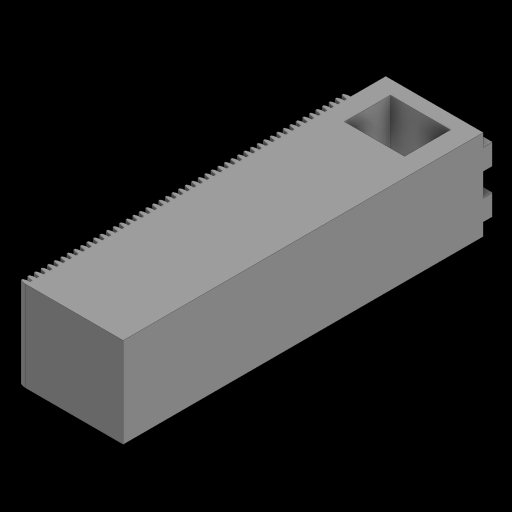
# Autodesk Inventor part: 렉기어
Saved by Autodesk Inventor 2023 (Build 270158000, 158)
## iProperties
Created: 2024-07-04
Part Number: 렉기어
Material: 일반
Document SubType Name: Modeling
Designer: OMS55
Density: 1 g/cm^3
Appearance: 기본값
Mass: 113.431 g
Surface Area: 254.945 cm^2
Volume: 113.431 cm^3
Author: OMS55
Autodesk Inventor part; units mm, degrees
ref_plane "YZ Plane" through (0, 0, 0) normal (1, 0, 0) x (0, 1, 0)
ref_plane "XZ Plane" through (0, 0, 0) normal (0, 1, 0) x (-1, 0, 0)
ref_plane "XY Plane" through (0, 0, 0) normal (0, 0, 1) x (1, 0, 0)
sketch "스케치1" plane through (0, 0, 0) normal (0, 1, 0) x (-1, 0, 0)
  line L0 (0, 0) -> (-34.5, 0)
  line L1 (-34.5, 0) -> (-34.5, -120)
  line L2 (-34.5, -120) -> (0, -120)
  line L3 (0, -120) -> (0, 0)
  line L4 (-2, 0) -> (-34.5, 0)
  line L5 (-34.5, 0) -> (-34.5, -120)
  line L6 (-34.5, -120) -> (-2, -120)
  line L7 (-2, -120) -> (-2, 0)
  arc A0 (0, -0.477) -> (-2, 0) centre (-2, -4.4314) ccw
  arc A1 (-2, -1.454) -> (0, -0.977) centre (-2, 2.9774) ccw
  line L8 (-2, -0.727) -> (0, -0.727) construction
  line L9 (0, -0.477) -> (0, -0.977)
  line L10 (-2, 0) -> (-2, -1.454)
  arc A2 (0, -2.658) -> (-2, -2.181) centre (-2, -6.6124) ccw
  line L11 (0, -2.658) -> (0, -3.158)
  arc A3 (-2, -3.635) -> (0, -3.158) centre (-2, 0.7964) ccw
  line L12 (-2, -2.181) -> (-2, -3.635)
  arc A4 (0, -4.839) -> (-2, -4.362) centre (-2, -8.7934) ccw
  line L13 (0, -4.839) -> (0, -5.339)
  arc A5 (-2, -5.816) -> (0, -5.339) centre (-2, -1.3846) ccw
  line L14 (-2, -4.362) -> (-2, -5.816)
  arc A6 (0, -7.02) -> (-2, -6.543) centre (-2, -10.9744) ccw
  line L15 (0, -7.02) -> (0, -7.52)
  arc A7 (-2, -7.997) -> (0, -7.52) centre (-2, -3.5656) ccw
  line L16 (-2, -6.543) -> (-2, -7.997)
  arc A8 (0, -9.201) -> (-2, -8.724) centre (-2, -13.1554) ccw
  line L17 (0, -9.201) -> (0, -9.701)
  arc A9 (-2, -10.178) -> (0, -9.701) centre (-2, -5.7466) ccw
  line L18 (-2, -8.724) -> (-2, -10.178)
  arc A10 (0, -11.382) -> (-2, -10.905) centre (-2, -15.3364) ccw
  line L19 (0, -11.382) -> (0, -11.882)
  arc A11 (-2, -12.359) -> (0, -11.882) centre (-2, -7.9276) ccw
  line L20 (-2, -10.905) -> (-2, -12.359)
  arc A12 (0, -13.563) -> (-2, -13.086) centre (-2, -17.5174) ccw
  line L21 (0, -13.563) -> (0, -14.063)
  arc A13 (-2, -14.54) -> (0, -14.063) centre (-2, -10.1086) ccw
  line L22 (-2, -13.086) -> (-2, -14.54)
  arc A14 (0, -15.744) -> (-2, -15.267) centre (-2, -19.6984) ccw
  line L23 (0, -15.744) -> (0, -16.244)
  arc A15 (-2, -16.721) -> (0, -16.244) centre (-2, -12.2896) ccw
  line L24 (-2, -15.267) -> (-2, -16.721)
  arc A16 (0, -17.925) -> (-2, -17.448) centre (-2, -21.8794) ccw
  line L25 (0, -17.925) -> (0, -18.425)
  arc A17 (-2, -18.902) -> (0, -18.425) centre (-2, -14.4706) ccw
  line L26 (-2, -17.448) -> (-2, -18.902)
  arc A18 (0, -20.106) -> (-2, -19.629) centre (-2, -24.0604) ccw
  line L27 (0, -20.106) -> (0, -20.606)
  arc A19 (-2, -21.083) -> (0, -20.606) centre (-2, -16.6516) ccw
  line L28 (-2, -19.629) -> (-2, -21.083)
  arc A20 (0, -22.287) -> (-2, -21.81) centre (-2, -26.2414) ccw
  line L29 (0, -22.287) -> (0, -22.787)
  arc A21 (-2, -23.264) -> (0, -22.787) centre (-2, -18.8326) ccw
  line L30 (-2, -21.81) -> (-2, -23.264)
  arc A22 (0, -24.468) -> (-2, -23.991) centre (-2, -28.4224) ccw
  line L31 (0, -24.468) -> (0, -24.968)
  arc A23 (-2, -25.445) -> (0, -24.968) centre (-2, -21.0136) ccw
  line L32 (-2, -23.991) -> (-2, -25.445)
  arc A24 (0, -26.649) -> (-2, -26.172) centre (-2, -30.6034) ccw
  line L33 (0, -26.649) -> (0, -27.149)
  arc A25 (-2, -27.626) -> (0, -27.149) centre (-2, -23.1946) ccw
  line L34 (-2, -26.172) -> (-2, -27.626)
  arc A26 (0, -28.83) -> (-2, -28.353) centre (-2, -32.7844) ccw
  line L35 (0, -28.83) -> (0, -29.33)
  arc A27 (-2, -29.807) -> (0, -29.33) centre (-2, -25.3756) ccw
  line L36 (-2, -28.353) -> (-2, -29.807)
  arc A28 (0, -31.011) -> (-2, -30.534) centre (-2, -34.9654) ccw
  line L37 (0, -31.011) -> (0, -31.511)
  arc A29 (-2, -31.988) -> (0, -31.511) centre (-2, -27.5566) ccw
  line L38 (-2, -30.534) -> (-2, -31.988)
  arc A30 (0, -33.192) -> (-2, -32.715) centre (-2, -37.1464) ccw
  line L39 (0, -33.192) -> (0, -33.692)
  arc A31 (-2, -34.169) -> (0, -33.692) centre (-2, -29.7376) ccw
  line L40 (-2, -32.715) -> (-2, -34.169)
  arc A32 (0, -35.373) -> (-2, -34.896) centre (-2, -39.3274) ccw
  line L41 (0, -35.373) -> (0, -35.873)
  arc A33 (-2, -36.35) -> (0, -35.873) centre (-2, -31.9186) ccw
  line L42 (-2, -34.896) -> (-2, -36.35)
  arc A34 (0, -37.554) -> (-2, -37.077) centre (-2, -41.5084) ccw
  line L43 (0, -37.554) -> (0, -38.054)
  arc A35 (-2, -38.531) -> (0, -38.054) centre (-2, -34.0996) ccw
  line L44 (-2, -37.077) -> (-2, -38.531)
  arc A36 (0, -39.735) -> (-2, -39.258) centre (-2, -43.6894) ccw
  line L45 (0, -39.735) -> (0, -40.235)
  arc A37 (-2, -40.712) -> (0, -40.235) centre (-2, -36.2806) ccw
  line L46 (-2, -39.258) -> (-2, -40.712)
  arc A38 (0, -41.916) -> (-2, -41.439) centre (-2, -45.8704) ccw
  line L47 (0, -41.916) -> (0, -42.416)
  arc A39 (-2, -42.893) -> (0, -42.416) centre (-2, -38.4616) ccw
  line L48 (-2, -41.439) -> (-2, -42.893)
  arc A40 (0, -44.097) -> (-2, -43.62) centre (-2, -48.0514) ccw
  line L49 (0, -44.097) -> (0, -44.597)
  arc A41 (-2, -45.074) -> (0, -44.597) centre (-2, -40.6426) ccw
  line L50 (-2, -43.62) -> (-2, -45.074)
  arc A42 (0, -46.278) -> (-2, -45.801) centre (-2, -50.2324) ccw
  line L51 (0, -46.278) -> (0, -46.778)
  arc A43 (-2, -47.255) -> (0, -46.778) centre (-2, -42.8236) ccw
  line L52 (-2, -45.801) -> (-2, -47.255)
  arc A44 (0, -48.459) -> (-2, -47.982) centre (-2, -52.4134) ccw
  line L53 (0, -48.459) -> (0, -48.959)
  arc A45 (-2, -49.436) -> (0, -48.959) centre (-2, -45.0046) ccw
  line L54 (-2, -47.982) -> (-2, -49.436)
  arc A46 (0, -50.64) -> (-2, -50.163) centre (-2, -54.5944) ccw
  line L55 (0, -50.64) -> (0, -51.14)
  arc A47 (-2, -51.617) -> (0, -51.14) centre (-2, -47.1856) ccw
  line L56 (-2, -50.163) -> (-2, -51.617)
  arc A48 (0, -52.821) -> (-2, -52.344) centre (-2, -56.7754) ccw
  line L57 (0, -52.821) -> (0, -53.321)
  arc A49 (-2, -53.798) -> (0, -53.321) centre (-2, -49.3666) ccw
  line L58 (-2, -52.344) -> (-2, -53.798)
  arc A50 (0, -55.002) -> (-2, -54.525) centre (-2, -58.9564) ccw
  line L59 (0, -55.002) -> (0, -55.502)
  arc A51 (-2, -55.979) -> (0, -55.502) centre (-2, -51.5476) ccw
  line L60 (-2, -54.525) -> (-2, -55.979)
  arc A52 (0, -57.183) -> (-2, -56.706) centre (-2, -61.1374) ccw
  line L61 (0, -57.183) -> (0, -57.683)
  arc A53 (-2, -58.16) -> (0, -57.683) centre (-2, -53.7286) ccw
  line L62 (-2, -56.706) -> (-2, -58.16)
  arc A54 (0, -59.364) -> (-2, -58.887) centre (-2, -63.3184) ccw
  line L63 (0, -59.364) -> (0, -59.864)
  arc A55 (-2, -60.341) -> (0, -59.864) centre (-2, -55.9096) ccw
  line L64 (-2, -58.887) -> (-2, -60.341)
  arc A56 (0, -61.545) -> (-2, -61.068) centre (-2, -65.4994) ccw
  line L65 (0, -61.545) -> (0, -62.045)
  arc A57 (-2, -62.522) -> (0, -62.045) centre (-2, -58.0906) ccw
  line L66 (-2, -61.068) -> (-2, -62.522)
  arc A58 (0, -63.726) -> (-2, -63.249) centre (-2, -67.6804) ccw
  line L67 (0, -63.726) -> (0, -64.226)
  arc A59 (-2, -64.703) -> (0, -64.226) centre (-2, -60.2716) ccw
  line L68 (-2, -63.249) -> (-2, -64.703)
  arc A60 (0, -65.907) -> (-2, -65.43) centre (-2, -69.8614) ccw
  line L69 (0, -65.907) -> (0, -66.407)
  arc A61 (-2, -66.884) -> (0, -66.407) centre (-2, -62.4526) ccw
  line L70 (-2, -65.43) -> (-2, -66.884)
  arc A62 (0, -68.088) -> (-2, -67.611) centre (-2, -72.0424) ccw
  line L71 (0, -68.088) -> (0, -68.588)
  arc A63 (-2, -69.065) -> (0, -68.588) centre (-2, -64.6336) ccw
  line L72 (-2, -67.611) -> (-2, -69.065)
  arc A64 (0, -70.269) -> (-2, -69.792) centre (-2, -74.2234) ccw
  line L73 (0, -70.269) -> (0, -70.769)
  arc A65 (-2, -71.246) -> (0, -70.769) centre (-2, -66.8146) ccw
  line L74 (-2, -69.792) -> (-2, -71.246)
  arc A66 (0, -72.45) -> (-2, -71.973) centre (-2, -76.4044) ccw
  line L75 (0, -72.45) -> (0, -72.95)
  arc A67 (-2, -73.427) -> (0, -72.95) centre (-2, -68.9956) ccw
  line L76 (-2, -71.973) -> (-2, -73.427)
  arc A68 (0, -74.631) -> (-2, -74.154) centre (-2, -78.5854) ccw
  line L77 (0, -74.631) -> (0, -75.131)
  arc A69 (-2, -75.608) -> (0, -75.131) centre (-2, -71.1766) ccw
  line L78 (-2, -74.154) -> (-2, -75.608)
  arc A70 (0, -76.812) -> (-2, -76.335) centre (-2, -80.7664) ccw
  line L79 (0, -76.812) -> (0, -77.312)
  arc A71 (-2, -77.789) -> (0, -77.312) centre (-2, -73.3576) ccw
  line L80 (-2, -76.335) -> (-2, -77.789)
  arc A72 (0, -78.993) -> (-2, -78.516) centre (-2, -82.9474) ccw
  line L81 (0, -78.993) -> (0, -79.493)
  arc A73 (-2, -79.97) -> (0, -79.493) centre (-2, -75.5386) ccw
  line L82 (-2, -78.516) -> (-2, -79.97)
  arc A74 (0, -81.174) -> (-2, -80.697) centre (-2, -85.1284) ccw
  line L83 (0, -81.174) -> (0, -81.674)
  arc A75 (-2, -82.151) -> (0, -81.674) centre (-2, -77.7196) ccw
  line L84 (-2, -80.697) -> (-2, -82.151)
  arc A76 (0, -83.355) -> (-2, -82.878) centre (-2, -87.3094) ccw
  line L85 (0, -83.355) -> (0, -83.855)
  arc A77 (-2, -84.332) -> (0, -83.855) centre (-2, -79.9006) ccw
  line L86 (-2, -82.878) -> (-2, -84.332)
  arc A78 (0, -85.536) -> (-2, -85.059) centre (-2, -89.4904) ccw
  line L87 (0, -85.536) -> (0, -86.036)
  arc A79 (-2, -86.513) -> (0, -86.036) centre (-2, -82.0816) ccw
  line L88 (-2, -85.059) -> (-2, -86.513)
  arc A80 (0, -87.717) -> (-2, -87.24) centre (-2, -91.6714) ccw
  line L89 (0, -87.717) -> (0, -88.217)
  arc A81 (-2, -88.694) -> (0, -88.217) centre (-2, -84.2626) ccw
  line L90 (-2, -87.24) -> (-2, -88.694)
  arc A82 (0, -89.898) -> (-2, -89.421) centre (-2, -93.8524) ccw
  line L91 (0, -89.898) -> (0, -90.398)
  arc A83 (-2, -90.875) -> (0, -90.398) centre (-2, -86.4436) ccw
  line L92 (-2, -89.421) -> (-2, -90.875)
  arc A84 (0, -92.079) -> (-2, -91.602) centre (-2, -96.0334) ccw
  line L93 (0, -92.079) -> (0, -92.579)
  arc A85 (-2, -93.056) -> (0, -92.579) centre (-2, -88.6246) ccw
  line L94 (-2, -91.602) -> (-2, -93.056)
  arc A86 (0, -94.26) -> (-2, -93.783) centre (-2, -98.2144) ccw
  line L95 (0, -94.26) -> (0, -94.76)
  arc A87 (-2, -95.237) -> (0, -94.76) centre (-2, -90.8056) ccw
  line L96 (-2, -93.783) -> (-2, -95.237)
  arc A88 (0, -96.441) -> (-2, -95.964) centre (-2, -100.3954) ccw
  line L97 (0, -96.441) -> (0, -96.941)
  arc A89 (-2, -97.418) -> (0, -96.941) centre (-2, -92.9866) ccw
  line L98 (-2, -95.964) -> (-2, -97.418)
  arc A90 (0, -98.622) -> (-2, -98.145) centre (-2, -102.5764) ccw
  line L99 (0, -98.622) -> (0, -99.122)
  arc A91 (-2, -99.599) -> (0, -99.122) centre (-2, -95.1676) ccw
  line L100 (-2, -98.145) -> (-2, -99.599)
  arc A92 (0, -100.803) -> (-2, -100.326) centre (-2, -104.7574) ccw
  line L101 (0, -100.803) -> (0, -101.303)
  arc A93 (-2, -101.78) -> (0, -101.303) centre (-2, -97.3486) ccw
  line L102 (-2, -100.326) -> (-2, -101.78)
  arc A94 (0, -102.984) -> (-2, -102.507) centre (-2, -106.9384) ccw
  line L103 (0, -102.984) -> (0, -103.484)
  arc A95 (-2, -103.961) -> (0, -103.484) centre (-2, -99.5296) ccw
  line L104 (-2, -102.507) -> (-2, -103.961)
  arc A96 (0, -105.165) -> (-2, -104.688) centre (-2, -109.1194) ccw
  line L105 (0, -105.165) -> (0, -105.665)
  arc A97 (-2, -106.142) -> (0, -105.665) centre (-2, -101.7106) ccw
  line L106 (-2, -104.688) -> (-2, -106.142)
  arc A98 (0, -107.346) -> (-2, -106.869) centre (-2, -111.3004) ccw
  line L107 (0, -107.346) -> (0, -107.846)
  arc A99 (-2, -108.323) -> (0, -107.846) centre (-2, -103.8916) ccw
  line L108 (-2, -106.869) -> (-2, -108.323)
  point P0 (-2, -84.332)
  point P1 (0, -83.355)
  point P2 (-2, -60.341)
  point P3 (0, -59.364)
  point P4 (-2, -58.887)
  point P5 (-2, -108.323)
  point P6 (0, -107.346)
  point P7 (-2, -106.142)
  point P8 (0, -105.165)
  point P9 (-2, -103.961)
  point P10 (0, -102.984)
  point P11 (-2, -101.78)
  point P12 (0, -100.803)
  point P13 (-2, -99.599)
  point P14 (0, -98.622)
  point P15 (-2, -97.418)
  point P16 (0, -96.441)
  point P17 (-2, -95.237)
  point P18 (0, -94.26)
  point P19 (-2, -93.056)
  point P20 (0, -92.079)
  point P21 (-2, -90.875)
  point P22 (0, -89.898)
  point P23 (0, -85.536)
  point P24 (-2, -88.694)
  point P25 (-2, -82.151)
  point P26 (0, -81.174)
  point P27 (-2, -79.97)
  point P28 (0, -78.993)
  point P29 (-2, -78.516)
  point P30 (-2, -77.789)
  point P31 (0, -76.812)
  point P32 (-2, -76.335)
  point P33 (-2, -75.608)
  point P34 (0, -74.631)
  point P35 (-2, -73.427)
  point P36 (0, -72.45)
  point P37 (-2, -71.246)
  point P38 (0, -70.269)
  point P39 (-2, -69.065)
  point P40 (0, -68.088)
  point P41 (-2, -66.884)
  point P42 (0, -65.907)
  point P43 (-2, -64.703)
  point P44 (0, -63.726)
  point P45 (-2, -63.249)
  point P46 (-2, -62.522)
  point P47 (0, -61.545)
  point P48 (-2, -61.068)
  point P49 (-2, -58.16)
  point P50 (0, -57.183)
  point P51 (-2, -56.706)
  point P52 (-2, -53.798)
  point P53 (0, -52.821)
  point P54 (-2, -52.344)
  point P55 (-2, -51.617)
  point P56 (0, -50.64)
  point P57 (-2, -50.163)
  point P58 (-2, -49.436)
  point P59 (0, -48.459)
  point P60 (-2, -47.982)
  point P61 (-2, -47.255)
  point P62 (0, -46.278)
  point P63 (-2, -45.801)
  point P64 (-2, -45.074)
  point P65 (0, -44.097)
  point P66 (-2, -43.62)
  point P67 (-2, -38.531)
  point P68 (0, -37.554)
  point P69 (-2, -34.169)
  point P70 (-2, -32.715)
  point P71 (-2, -29.807)
  point P72 (0, -28.83)
  point P73 (-2, -28.353)
  point P74 (-2, -25.445)
  point P75 (0, -24.468)
  point P76 (-2, -23.991)
  point P77 (-2, -23.264)
  point P78 (0, -22.287)
  point P79 (-2, -21.81)
  point P80 (-2, -55.979)
  point P81 (0, -55.002)
  point P82 (-2, -54.525)
  point P83 (-2, -42.893)
  point P84 (0, -41.916)
  point P85 (-2, -41.439)
  point P86 (-2, -40.712)
  point P87 (0, -39.735)
  point P88 (-2, -39.258)
  point P89 (-2, -36.35)
  point P90 (0, -35.373)
  point P91 (-2, -31.988)
  point P92 (-2, -30.534)
  point P93 (-2, -27.626)
  point P94 (0, -26.649)
  point P95 (-2, -26.172)
  point P96 (-2, -21.083)
  point P97 (0, -20.106)
  point P98 (-2, -19.629)
  point P99 (-2, -18.902)
  point P100 (-2, -16.721)
  point P101 (-2, -14.54)
  point P102 (0, -13.563)
  point P103 (-2, -12.359)
  point P104 (0, -11.382)
  point P105 (-2, -10.178)
  point P106 (-2, -7.997)
  point P107 (0, -7.02)
  point P108 (-2, -5.816)
  point P109 (0, -4.839)
  point P110 (-2, -4.362)
  point P111 (-2, -3.635)
  point P112 (0, -2.658)
  point P113 (-2, -2.181)
  point P114 (0, -87.717)
  point P115 (-2, -86.513)
  dimension "d0" = 120
  dimension "d1" = 34.5
  dimension "d2" = 120
  dimension "d3" = 32.5
  dimension "d4" = 1.454
  dimension "d7" = 0.727
  dimension "d8" = 0.25
  dimension "d9" = 0.25
  dimension "d14" = 2.181
  constraints: 294 vertical alignment, 214 end point, 200 point on circle, 100 centre point, 98 collinear, 98 equal radius, 4 vertical, 3 horizontal, 2 parallel, 2 perpendicular, 1 coincident, 1 tangent, 10 other
  measures "d0" distance of L2.end L0.start
  measures "d1" distance of L0.start L0.end
  measures "d2" distance of L6.end L4.start
  measures "d3" distance of L0.end L4.start
  measures "d4" distance of L10.end L4.start
  measures "d7" distance of L8.start L4.start
  measures "d8" distance of L8.end L9.start
  measures "d9" distance of L8.end L9.end
  measures "d14" distance of A0.centre A2.centre
extrude "돌출1" add sketch "스케치1" along normal blind 30 contours L7 L2 L1 L0 | A0 L3 A1 L7 | A2 L3 A3 L7 | L7 A98 L3 A99 | A4 L3 A5 L7 | L7 A96 L3 A97 | A6 L3 A7 L7 | L7 A94 L3 A95 | A8 L3 A9 L7 | L7 A92 L3 A93 | A10 L3 A11 L7 | L7 A90 L3 A91 | A12 L3 A13 L7 | L7 A88 L3 A89 | A14 L3 A15 L7 | L7 A86 L3 A87 | A16 L3 A17 L7 | L7 A84 L3 A85 | A18 L3 A19 L7 | L7 A82 L3 A83 | A20 L3 A21 L7 | L7 A80 L3 A81 | A22 L3 A23 L7 | L7 A79 L3 A80 | L7 A78 L3 A79 | A24 L3 A25 L7 | L7 A76 L3 A77 | A26 L3 A27 L7 | L7 A74 L3 A75 | A28 L3 A29 L7 | L7 A72 L3 A73 | A30 L3 A31 L7 | L7 A70 L3 A71 | A32 L3 A33 L7 | L7 A68 L3 A69 | A34 L3 A35 L7 | L7 A66 L3 A67 | A36 L3 A37 L7 | L7 A64 L3 A65 | A38 L3 A39 L7 | L7 A62 L3 A63 | A40 L3 A41 L7 | L7 A60 L3 A61 | A42 L3 A43 L7 | L7 A58 L3 A59 | A44 L3 A45 L7 | L7 A56 L3 A57 | A46 L3 A47 L7 | L7 A54 L3 A55 | A48 L3 A49 L7 | L7 A52 L3 A53 | A50 L3 A51 L7
extrude "돌출2" cut sketch "스케치1" along normal blind 30 contours L7 A79 L3 A80
sketch "스케치2" plane through (34.5, 0, -120) normal (0, 0, -1) x (-1, 0, 0)
  line L0 (32.5, 25.8) -> (0, 25.8)
  line L1 (0, 25.8) -> (0, 18.8)
  line L2 (0, 18.8) -> (32.5, 18.8)
  line L3 (32.5, 18.8) -> (32.5, 25.8)
  line L4 (32.5, 11.2) -> (0, 11.2)
  line L5 (0, 11.2) -> (0, 4.2)
  line L6 (0, 4.2) -> (32.5, 4.2)
  line L7 (32.5, 4.2) -> (32.5, 11.2)
  line L8 (32.5, 18.8) -> (32.5, 11.2) construction
  line L9 (0, 18.8) -> (0, 11.2) construction
  line L10 (32.5, 0) -> (32.5, 30) construction
  line L11 (0, 0) -> (0, 30) construction
  point P0 (34.5, 0)
  point P1 (32.5, 15)
  point P2 (32.5, 15)
  dimension "d21" = 7.6
  dimension "d22" = 7
  dimension "d23" = 7
  constraints: 20 end point, 5 parallel, 2 collinear, 2 horizontal, 2 midpoint, 2 perpendicular, 2 point on line, 1 coincident, 1 vertical
  measures "d21" distance between parallel lines of L4 L2
  measures "d22" distance of L2.end L0.start
  measures "d23" distance of L6.end L4.start
extrude "돌출3" add sketch "스케치2" along normal blind 3
sketch "스케치4" plane through (0, 30, 0) normal (0, 1, 0) x (1, 0, 0)
  line L0 (28.25, 115.3) -> (8.25, 115.3)
  line L1 (8.25, 115.3) -> (8.25, 100)
  line L2 (8.25, 100) -> (28.25, 100)
  line L3 (28.25, 100) -> (28.25, 115.3)
  line L4 (34.5, 120) -> (2, 120) projected
  line L5 (34.5, 0) -> (34.5, 120) projected
  point P0 (0, 0)
  dimension "d26" = 20
  dimension "d27" = 20
  dimension "d28" = 6.25
  dimension "d29" = 4.7
  constraints: 8 end point, 2 parallel, 1 horizontal, 1 perpendicular
  measures "d26" distance between parallel lines of L2 L4
  measures "d27" distance between parallel lines of L1 L3
  measures "d28" distance between parallel lines of L5 L3
  measures "d29" distance between parallel lines of L4 L0
extrude "돌출4" cut sketch "스케치4" against normal blind 30
sketch "스케치5" plane through (8.25, 30, -115.3) normal (0, 0, 1) x (1, 0, 0)
  circle A0 centre (7.45, -15) radius 1.45
  line L0 (-6.25, -18.8) -> (-6.25, -11.2) projected
  point P0 (-8.25, -30)
  point P1 (-6.25, -15)
  dimension "d33" = 13.7
  constraints: 1 centre point, 1 horizontal alignment, 1 midpoint
  measures "d33" distance from line of L0 A0.centre
extrude "돌출5" cut sketch "스케치5" against normal blind 30
